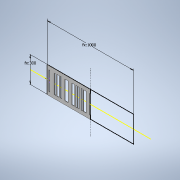
# Autodesk Inventor part: ferrite_layer_dex_0R2
Saved by Autodesk Inventor 2021 (Build 250183000, 183)
## iProperties
Created: 2021-01-27
Part Number: ferrite_layer_dex_0R2
Material: Generic
Document SubType Name: Modeling
Designer: pduy110
Density: 1 g/cm^3
Appearance: Default
Author: pduy110
Autodesk Inventor part; units mm, degrees
ref_plane "YZ Plane" through (0, 0, 0) normal (1, 0, 0) x (0, 1, 0)
ref_plane "XZ Plane" through (0, 0, 0) normal (0, 1, 0) x (-1, 0, 0)
ref_plane "XY Plane" through (0, 0, 0) normal (0, 0, 1) x (1, 0, 0)
sketch "ferrite_layer_outline_sketch" plane through (0, 0, 0) normal (0, 0, 1) x (1, 0, 0)
  line L0 (0, 150) -> (1000, 150)
  line L1 (1000, 150) -> (1000, -150)
  line L2 (1000, -150) -> (0, -150)
  line L3 (0, -150) -> (0, 150)
  line L4 (-200, 0) -> (1200, 0) projected
  line L5 (500, 150) -> (500, -150) construction
  line L6 (500, 366.8869) -> (500, -324.3455) construction
  line L7 (500, 150) -> (500, -150)
  point P0 (0, 0)
  point P1 (0, 0)
  point P2 (0, 0)
  point P3 (0, 0)
  point P4 (20, 0)
  dimension "d0" = 1000
  dimension "d1" = 300
  constraints: 14 end point, 3 coincident, 3 midpoint, 3 point on line, 2 parallel, 1 collinear, 1 horizontal, 1 perpendicular
  measures "d0" distance between parallel lines of L1 L3
  measures "d1" distance between parallel lines of L2 L0
extrude "Extrusion8" add sketch "ferrite_layer_outline_sketch" along normal blind 4 contours L0 L7 L4 L3 | L4 L7 L2 L3
ref_plane "acrylic_sheet_plane" through (0, 0, 4) normal (0, 0, 1) x (1, 0, 0)
sketch "Sketch4" plane through (0, 0, 4) normal (0, 0, 1) x (1, 0, 0)
  line L0 (20, 109) -> (35, 109)
  line L1 (35, 109) -> (35, -109)
  line L2 (35, -109) -> (20, -109)
  line L3 (20, -109) -> (20, 109)
  line L4 (-12.6534, 0) -> (47.471, 0)
  line L5 (0, 150) -> (0, -150) projected
  line L6 (500, 150) -> (0, 150) projected
  line L7 (0, -150) -> (500, -150) projected
  point P0 (0, 0)
  point P1 (20, 0)
  point P2 (0, 0)
  point P3 (1000, 150)
  point P4 (1000, -150)
  dimension "d43" = 15
  dimension "d44" = 218
  dimension "d45" = 20
  constraints: 12 end point, 2 horizontal, 2 midpoint, 2 parallel, 2 point on line, 1 perpendicular
  measures "d43" distance between parallel lines of L1 L3
  measures "d44" distance between parallel lines of L2 L0
  measures "d45" distance between parallel lines of L5 L3
extrude "Extrusion9" cut sketch "Sketch4" against normal through all
pattern_linear "Rectangular Pattern 11 fer" count 11 spacing 94.5 along (1, 0, 0) of "Extrusion9"
pattern_linear "Rectangular Pattern 8 fer" count 8 spacing 135 along (1, 0, 0) of "Extrusion9"
pattern_linear "Rectangular Pattern 10 fer" count 10 spacing 105 along (1, 0, 0) of "Extrusion9"
pattern_linear "pattern_test_#_of_ferrites 15 fer" count 15 spacing 67.5 along (1, 0, 0) of "Extrusion9"
equation "\"d0\" = track_length"
equation "\"d1\" = track_width"
equation "\"d43\" = ferrite_width"
equation "\"d44\" = ferrite_length"
equation "\"d45\" = gap_distance"
equation "\"d50\" = parameter_5"
equation "\"d62\" = test_parameter_5"
equation "\"track_length\" = 1000"
equation "\"track_width\" = 300"
equation "\"gap_distance\" = 20"
equation "\"ferrite_length\" = 218"
equation "\"ferrite_width\" = 15"
equation "\"ferrite_height\" = 8"
equation "\"acrylic_sheet_8mm\" = 8"
equation "\"parameter_5\" = 94.5"
equation "\"test_parameter_5\" = 67.5"
body "Solid8"
